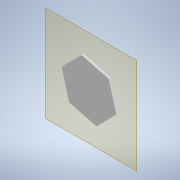
# Autodesk Inventor part: Part9
Saved by Autodesk Inventor 2020 (Build 240168000, 168)
## iProperties
Created: 2022-04-27
Part Number: Part9
Material: Generic
Document SubType Name: Modeling
Designer: Manish
Density: 1 g/cm^3
Appearance: Default
Author: Manish
Autodesk Inventor part; units mm, degrees
ref_plane "YZ Plane" through (0, 0, 0) normal (1, 0, 0) x (0, 1, 0)
ref_plane "XZ Plane" through (0, 0, 0) normal (0, 1, 0) x (-1, 0, 0)
ref_plane "XY Plane" through (0, 0, 0) normal (0, 0, 1) x (1, 0, 0)
ref_plane "Work Plane1" through (0, 791.1285, 0) normal (0, 0, 1) x (1, 0, 0)
sketch "Sketch1" plane through (0, 791.1285, 0) normal (0, 0, 1) x (1, 0, 0)
  line L0 (328.4462, -876.9707) -> (81.1956, -1128.3595)
  line L1 (81.1956, -1128.3595) -> (112.918, -1159.5597)
  line L2 (112.918, -1159.5597) -> (360.1686, -908.1709)
  line L3 (360.1686, -908.1709) -> (328.4462, -876.9707)
  line L4 (259.0451, -532.0835) -> (0, -791.1285)
  line L5 (0, -791.1285) -> (-263.229, -1054.3575)
  line L6 (-85.8422, -462.6823) -> (-337.231, -709.9329)
  line L7 (-337.231, -709.9329) -> (-368.4312, -678.2105)
  line L8 (-368.4312, -678.2105) -> (-117.0424, -430.9599)
  line L9 (-117.0424, -430.9599) -> (-85.8422, -462.6823)
  line L10 (237.1469, -307.0605) -> (-387.5175, -931.7249)
  line L11 (375.5297, -877.5543) -> (281.446, -537.7346)
  line L12 (238.5647, -549.6068) -> (332.6484, -889.4265)
  line L13 (281.446, -537.7346) -> (238.5647, -549.6068)
  line L14 (332.6484, -889.4265) -> (375.5297, -877.5543)
  line L15 (262.6118, -509.1231) -> (-78.7226, -420.6921)
  line L16 (-89.8816, -463.7646) -> (251.4528, -552.1956)
  line L17 (-78.7226, -420.6921) -> (-89.8816, -463.7646)
  line L18 (251.4528, -552.1956) -> (262.6118, -509.1231)
  line L19 (-112.918, -422.6973) -> (-360.1686, -674.0861)
  line L20 (-328.4462, -705.2863) -> (-81.1956, -453.8975)
  line L21 (-360.1686, -674.0861) -> (-328.4462, -705.2863)
  line L22 (-81.1956, -453.8975) -> (-112.918, -422.6973)
  line L23 (-375.5297, -704.7028) -> (-281.446, -1044.5225)
  line L24 (-238.5647, -1032.6502) -> (-332.6484, -692.8305)
  line L25 (-281.446, -1044.5225) -> (-238.5647, -1032.6502)
  line L26 (-332.6484, -692.8305) -> (-375.5297, -704.7028)
  line L27 (-262.6118, -1073.134) -> (78.7226, -1161.5649)
  line L28 (89.8816, -1118.4924) -> (-251.4528, -1030.0615)
  line L29 (78.7226, -1161.5649) -> (89.8816, -1118.4924)
  line L30 (-251.4528, -1030.0615) -> (-262.6118, -1073.134)
  point P0 (-329.4818, -704.2678)
  point P1 (-239.9645, -1033.0378)
  point P2 (89.5173, -1119.8985)
  point P3 (329.4818, -877.9893)
  point P4 (239.9645, -549.2193)
  point P5 (-87.5554, -464.3673)
  point P6 (-208.1509, -582.9776)
  dimension "d0" = 174.5996
  dimension "d1" = 0.475
  dimension "d2" = 352.6034
  dimension "d5" = 360
  constraints: 62 end point, 7 point on line, 5 symmetric about line, 3 parallel, 1 perpendicular, 55 other
  measures "d0" distance between parallel lines of L4 L10
  measures "d1" angle of L6 L10
  measures "d2" distance between parallel lines of L1 L3
extrude "Extrusion1" add sketch "Sketch1" along normal blind 25.4 contours L0 L29 L28 L25 L24 L5 L4 L12 L3 | L4 L5 L24 L10 L16 L13 L12 | L10 L24 L21 L20 L6 L16
body "Solid1"
